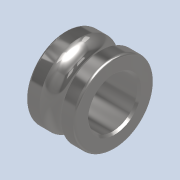
# Autodesk Inventor part: 040205DR-19-H6_ir
Saved by Autodesk Inventor 2021.2 (Build 252289000, 289)
## iProperties
Category: PARTsolutions
Company: TOKBEARING
Part Number: 040205DR-19-H6_ir
Material: 鉄、鋳鉄
Catalog Web Link: www.cadenas.de
Description: DR-H ir-D-Series bearings
Vendor: TOKBEARING
Document SubType Name: Modeling
Designer: partserver
Manufacturer: TOKBEARING
Mass: 8100 g
Surface Area: 3.80929 cm^2
Volume: 0.230488 cm^3
Density: 7.15 g/cm^3
Appearance: 半つや出し
PSOL_IDENT_0: {$CADENAS_DATA\23d-libs\tok_bearing\d_series_bearings\dr_h\dr_h_ir.prj},177 {VTYP=3D},{NB=040205DR-1
PSOL_IDENT_1: 9-H6_ir},{LINA=040205DR-19-H6_ir},{NN=DR-H ir},{DATE=16.12.2020 00:38:04},{GEOMDATE=19.02.2013 00:00
PSOL_IDENT_2: :00},{VERSION=},{LINEID=1520},{WBVAR=},{WBNUMERIC=}  {NB=040205DR-19-H6_ir},{LINA=040205DR-19-H6_ir}
PSOL_IDENT_3: ,{KT=DUMMY},{IDNR=},{CODE=040205},{PN=DR-19-H6},{D=19},{SD=6.0},{W=6.0},{W1=-},{W1X=0.000},{W2=-},{W
PSOL_IDENT_4: 2X=0.000},{LOAD=49 (5)},{TYPE=10},{QTY=2.500},{GW=8.1},{BD=3.06},{OP=35.2622},{N=5},{R=5.615},{GP=3.
PSOL_IDENT_5: 12}
NB: 040205DR-19-H6_ir
NN: DR-H ir
NT: D-Series bearings
NBSYN: $CODE.$PN._ir
LINA: 040205DR-19-H6_ir
CATALOG: TOK, Inc
CODE: 040205
PN: DR-19-H6
D: 19
SD: 6
W: 6
W1: -
W2: -
LOAD: 49 (5)
TYPE: 10
QTY: 2.500
GW: 8.1
SUPPLIER: TOKBEARING
ARTICLENO: 040205DR-19-H6_ir
BOMINFO: 040205DR-19-H6_ir
CREATOR: CADENAS GmbH
Title: 040205DR-19-H6_ir
Author: Cadenas PARTsolutions
Comments: D-Series bearings
Autodesk Inventor part; units mm, degrees
sketch "Sketch_2" plane through (0, 0, 0) normal (0, 0, 1) x (1, 0, 0)
  line L0 (6, 0) -> (0, 0)
  line L1 (0, 3.24) -> (0.24, 3)
  line L2 (0.24, 3) -> (5.76, 3)
  line L3 (5.76, 3) -> (6, 3.24)
  line L4 (6, 3.24) -> (6, 4.55)
  arc A0 (6, 4.55) -> (5.7, 4.85) centre (5.7, 4.55) ccw
  line L5 (5.7, 4.85) -> (4.325, 4.85)
  arc A1 (1.675, 4.85) -> (4.325, 4.85) centre (3, 5.615) ccw
  line L6 (1.675, 4.85) -> (0.3, 4.85)
  arc A2 (0.3, 4.85) -> (0, 4.55) centre (0.3, 4.55) ccw
  line L7 (0, 4.55) -> (0, 3.24)
  constraints: 16 end point, 6 point on circle, 3 centre point
revolve "Revolution1" add sketch "Sketch_2" angle 360 about axis through (6, 0, 0) along (1, 0, 0)
ref_plane "Dummy_IR_XY" through (0, 0, 0) normal (1, 0, 0) x (0, 0, -1)
ref_plane "Dummy_IR_YZ" through (0, 0, 0) normal (0, 0, -1) x (0, 1, 0)
ref_plane "Dummy_IR_ZX" through (0, 0, 0) normal (0, 1, 0) x (1, 0, 0)
ref_plane "IR_OR_XY" through (0, 0, 0) normal (1, 0, 0) x (0, 0, -1)
ref_plane "IR_OR_YZ" through (0, 0, 0) normal (0, 0, -1) x (0, 1, 0)
ref_plane "IR_OR_ZX" through (0, 0, 0) normal (0, 1, 0) x (1, 0, 0)
body "Solid1"
